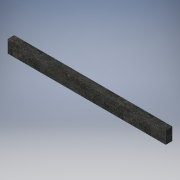
# Autodesk Inventor part: Steel support
Saved by Autodesk Inventor 2019 (Build 230136000, 136)
## iProperties
Created: 2021-03-08
Part Number: Steel support
Material: Steel
Document SubType Name: Modeling
Designer: User
Density: 7.85 g/cm^3
Appearance: Plate
Author: User
Autodesk Inventor part; units mm, degrees
ref_plane "YZ Plane" through (0, 0, 0) normal (1, 0, 0) x (0, 1, 0)
ref_plane "XZ Plane" through (0, 0, 0) normal (0, 1, 0) x (-1, 0, 0)
ref_plane "XY Plane" through (0, 0, 0) normal (0, 0, 1) x (1, 0, 0)
sketch "Sketch1" plane through (0, 0, 0) normal (0, 0, 1) x (1, 0, 0)
  line L0 (-32.3543, 10) -> (217.6457, 10)
  line L1 (217.6457, 10) -> (217.6457, -10)
  line L2 (217.6457, -10) -> (-32.3543, -10)
  line L3 (-32.3543, -10) -> (-32.3543, 10)
  point P0 (0, 0)
  dimension "d0" = 250
  dimension "d1" = 20
  dimension "d2" = 217.6457
  dimension "d3" = 10
  constraints: 8 end point, 2 parallel, 1 horizontal, 1 perpendicular
  measures "d0" distance between parallel lines of L1 L3
  measures "d1" distance between parallel lines of L0 L2
  measures "d2" distance from line of point (0, 0) L1
  measures "d3" distance from line of point (0, 0) L0
extrude "Extrusion1" add sketch "Sketch1" along normal mid plane 10
body "Solid1"
